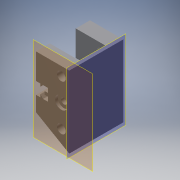
# Autodesk Inventor part: Z Slide
Saved by Autodesk Inventor 2016 (Build 200138000, 138)
## iProperties
Created: 2016-04-10
Part Number: Z Slide
Material: Generic
Document SubType Name: Modeling
Designer: Scott
Density: 1 g/cm^3
Appearance: Default
Author: Scott
Autodesk Inventor part; units mm, degrees
ref_plane "YZ Plane" through (0, 0, 0) normal (1, 0, 0) x (0, 1, 0)
ref_plane "XZ Plane" through (0, 0, 0) normal (0, 1, 0) x (-1, 0, 0)
ref_plane "XY Plane" through (0, 0, 0) normal (0, 0, 1) x (1, 0, 0)
ref_plane "Work Plane1" through (-126.0319, -64.0311, -0.0006) normal (-1, 0, 0) x (0, -1, 0)
ref_plane "Work Plane2" through (-119.6819, 11.1706, 49.5294) normal (0, 0, 1) x (0, 1, 0)
sketch "Sketch1" plane through (-119.6819, 11.1706, 49.5294) normal (0, 0, 1) x (0, 1, 0)
  line L0 (-9.2697, 67.31) -> (-9.2697, 6.35) projected
  line L1 (-9.2697, 6.35) -> (-141.1337, 6.35) projected
  line L2 (-141.1337, 6.35) -> (-141.1337, -31.75) projected
  line L3 (0, -31.75) -> (-141.1337, -31.75) projected
  line L4 (0, -31.75) -> (0, 67.31) projected
  line L5 (-9.2697, 67.31) -> (0, 67.31) projected
  line L6 (-141.1337, 6.35) -> (-105.9385, 67.31)
  line L7 (-141.1337, 6.35) -> (-70.7432, 6.35) construction
  line L8 (-105.9385, 67.31) -> (-9.2697, 67.31)
  point P0 (-11.1706, -119.6819)
  dimension "d0" = 60
  constraints: 6 end point, 2 horizontal, 1 equal length
  measures "d0" angle of L7 L6
ref_plane "Work Plane3" through (-186.9919, -129.9631, -49.5306) normal (0, 0, -1) x (0, 1, 0)
extrude "Extrusion1" add sketch "Sketch1" against normal up to surface (99.06 mm away) contours L0 L1 L6 L8
sketch "Sketch2" plane through (-186.9919, 1.9009, 49.5294) normal (0, 1, 0) x (1, 0, 0)
  line L0 (60.96, 0) -> (60.96, 99.06) projected
  line L1 (60.96, 25.3405) -> (-40.4029, 25.3405)
  line L2 (-40.4029, 25.3405) -> (-40.4029, 72.9974)
  line L3 (-40.4029, 72.9974) -> (60.96, 72.9974)
  line L4 (60.96, 72.9974) -> (60.96, 25.3405)
  point P0 (186.9919, 49.5294)
  constraints: 8 end point, 2 parallel, 1 horizontal, 1 perpendicular, 1 point on line
extrude "Extrusion2" cut sketch "Sketch2" against normal blind 61.9125
sketch "Sketch3" plane through (-119.6819, 11.1706, 49.5294) normal (0, 0, 1) x (1, 0, 0)
  line L0 (-67.31, -9.2697) -> (-67.31, -105.9385) projected
  line L1 (-67.31, -105.9385) -> (-6.35, -141.1337) projected
  line L2 (-6.35, -141.1337) -> (-6.35, -9.2697) projected
  line L3 (-6.35, -9.2697) -> (-67.31, -9.2697) projected
  circle A0 centre (-20.8167, -25.4098) radius 8
  circle A1 centre (-20.8167, -109.1654) radius 8
  line L4 (-20.8167, -25.4098) -> (-20.8167, -109.1654)
  circle A2 centre (-20.8167, -67.2876) radius 5.5
  point P0 (119.6819, -11.1706)
  dimension "d5" = 16
  dimension "d6" = 16
  dimension "d7" = 11
  constraints: 3 centre point, 2 end point, 1 midpoint, 1 vertical
  measures "d5" diameter of A0
  measures "d6" diameter of A1
  measures "d7" diameter of A2
extrude "Extrusion3" cut sketch "Sketch3" against normal blind 227.0125 contours A0 | A1 | A2 L4 | L4 A2
sketch "Sketch4" plane through (-119.6819, 11.1706, 49.5294) normal (0, 0, 1) x (1, 0, 0)
  arc A0 (-16.9332, -71.1822) -> (-24.7003, -71.1822) centre (-20.8167, -67.2876) ccw projected
  circle A1 centre (-20.8167, -67.2876) radius 11.5
  point P0 (119.6819, -11.1706)
  dimension "d10" = 23
  constraints: 1 centre point, 1 coincident
  measures "d10" diameter of A1
extrude "Extrusion4" cut sketch "Sketch4" against normal blind 5
sketch "Sketch5" plane through (-186.9919, -94.7679, 49.5294) normal (-1, 0, 0) x (0, 0, 1)
  line L0 (0, 0) -> (-99.06, 0) projected
  line L1 (-72.9974, 34.7562) -> (-72.9974, 96.6687) projected
  line L2 (-72.9974, 96.6687) -> (-99.06, 96.6687) projected
  line L3 (-99.06, 96.6687) -> (-99.06, 0) projected
  line L4 (0, 0) -> (-99.06, 0) projected
  line L5 (0, 96.6687) -> (0, 0) projected
  line L6 (0, 96.6687) -> (-25.3405, 96.6687) projected
  line L7 (-25.3405, 96.6687) -> (-25.3405, 34.7562) projected
  line L8 (-25.3405, 34.7562) -> (-72.9974, 34.7562) projected
  line L9 (-25.3405, 34.7562) -> (-25.3405, 44.1509) projected
  line L10 (-25.3405, 34.7562) -> (-72.9974, 34.7562)
  line L11 (-72.9974, 34.7562) -> (-72.9974, 22.0562)
  line L12 (-72.9974, 22.0562) -> (-25.3405, 22.0562)
  line L13 (-25.3405, 22.0562) -> (-25.3405, 34.7562)
  point P0 (-49.5294, 94.7679)
  dimension "d13" = 12.7
  constraints: 8 end point, 2 parallel, 1 horizontal, 1 perpendicular
  measures "d13" distance of L11.end L10.end
ref_plane "Work Plane4" through (-126.0319, -129.9631, -49.5306) normal (-1, 0, 0) x (0, 0, 1)
extrude "Extrusion5" cut sketch "Sketch5" against normal up to surface (60.96 mm away) contours L8 L13 L12 L11
sketch "Sketch6" plane through (-126.0319, -129.9631, 49.5294) normal (1, 0, 0) x (0, 0, -1)
  line L0 (72.9974, 57.2515) -> (72.9974, 131.864) projected
  line L1 (72.9974, 131.864) -> (99.06, 131.864) projected
  line L2 (99.06, 131.864) -> (99.06, 35.1953) projected
  line L3 (0, 35.1953) -> (99.06, 35.1953) projected
  line L4 (0, 131.864) -> (0, 35.1953) projected
  line L5 (0, 131.864) -> (25.3405, 131.864) projected
  line L6 (25.3405, 131.864) -> (25.3405, 57.2515) projected
  line L7 (25.3405, 57.2515) -> (72.9974, 57.2515) projected
  line L8 (72.9974, 131.864) -> (72.9974, 57.2515) projected
  line L9 (72.9974, 57.2515) -> (25.3405, 57.2515)
  line L10 (25.3405, 57.2515) -> (25.3405, 131.864)
  line L11 (25.3405, 131.864) -> (72.9974, 131.864)
  line L12 (72.9974, 131.864) -> (72.9974, 57.2515)
  point P0 (49.5294, 129.9631)
  constraints: 8 end point, 2 parallel, 1 horizontal, 1 perpendicular
extrude "Extrusion6" add sketch "Sketch6" against normal blind 7 contours L7 L6 L11 L0
sketch "Sketch7" plane through (-119.6819, 11.1706, 49.5294) normal (0, 0, 1) x (1, 0, 0)
  circle A0 centre (-20.8167, -67.2876) radius 11.5 projected
  circle A1 centre (-20.8167, -25.4098) radius 8 projected
  circle A2 centre (-20.8167, -109.1654) radius 8 projected
  line L0 (-67.31, -9.2697) -> (-67.31, -105.9385) projected
  line L1 (-67.31, -105.9385) -> (-6.35, -141.1337) projected
  line L2 (-6.35, -141.1337) -> (-6.35, -9.2697) projected
  line L3 (-6.35, -9.2697) -> (-67.31, -9.2697) projected
  line L4 (-45.32, -56.2876) -> (-67.32, -56.2876)
  line L5 (-67.32, -56.2876) -> (-67.32, -78.2876)
  line L6 (-67.32, -78.2876) -> (-45.32, -78.2876)
  line L7 (-45.32, -78.2876) -> (-45.32, -56.2876)
  line L8 (-45.32, -56.2876) -> (-67.32, -78.2876) construction
  line L9 (-67.32, -56.2876) -> (-45.32, -78.2876) construction
  point P0 (119.6819, -11.1706)
  point P1 (-56.32, -67.2876)
  dimension "d18" = 22
  dimension "d19" = 22
  constraints: 12 end point, 2 midpoint, 2 parallel, 1 horizontal, 1 perpendicular
  measures "d18" distance of L6.end L5.end
  measures "d19" distance of L5.end L4.end
extrude "Extrusion7" cut sketch "Sketch7" against normal blind 508 contours L4 L7 L6 L0 | L0 L6 L5 L4
sketch "Sketch8" plane through (-119.6819, 11.1706, 49.5294) normal (0, 0, 1) x (1, 0, 0)
  line L0 (-67.31, -56.2876) -> (-45.32, -56.2876) projected
  line L1 (-45.32, -56.2876) -> (-45.32, -78.2876) projected
  line L2 (-45.32, -78.2876) -> (-67.31, -78.2876) projected
  line L3 (-67.31, -78.2876) -> (-67.31, -105.9385) projected
  line L4 (-67.31, -105.9385) -> (-6.35, -141.1337) projected
  line L5 (-6.35, -141.1337) -> (-6.35, -9.2697) projected
  line L6 (-6.35, -9.2697) -> (-67.31, -9.2697) projected
  line L7 (-67.31, -9.2697) -> (-67.31, -56.2876) projected
  circle A0 centre (-20.8167, -109.1654) radius 8 projected
  circle A1 centre (-20.8167, -25.4098) radius 8 projected
  circle A2 centre (-20.8167, -67.2876) radius 11.5 projected
  line L8 (-45.32, -67.2876) -> (-48.32, -67.2876)
  line L9 (-51.32, -64.2876) -> (-45.32, -64.2876)
  line L10 (-45.32, -64.2876) -> (-45.32, -70.2876)
  line L11 (-45.32, -70.2876) -> (-51.32, -70.2876)
  line L12 (-51.32, -70.2876) -> (-51.32, -64.2876)
  line L13 (-51.32, -64.2876) -> (-45.32, -70.2876) construction
  line L14 (-45.32, -64.2876) -> (-51.32, -70.2876) construction
  line L15 (-45.32, -78.2876) -> (-45.32, -56.2876) projected
  line L16 (-45.32, -78.2876) -> (-56.315, -78.2876)
  line L17 (-67.31, -78.2876) -> (-45.32, -78.2876) projected
  line L18 (-56.315, -78.2876) -> (-59.315, -78.2876)
  line L19 (-59.315, -78.2876) -> (-59.315, -73.2876)
  line L20 (-59.315, -73.2876) -> (-54.315, -78.2876)
  line L21 (-59.315, -56.2876) -> (-59.315, -61.2876)
  line L22 (-59.315, -61.2876) -> (-54.315, -56.2876)
  line L23 (-45.32, -56.2876) -> (-67.31, -56.2876) projected
  line L24 (-59.315, -56.2876) -> (-54.315, -56.2876)
  point P0 (119.6819, -11.1706)
  dimension "d22" = 3
  dimension "d23" = 6
  dimension "d24" = 6
  dimension "d25" = 3
  dimension "d26" = 5
  dimension "d27" = 5
  constraints: 28 end point, 4 midpoint, 4 point on line, 2 horizontal, 2 parallel, 2 perpendicular, 1 collinear, 1 vertical
  measures "d22" distance of L8.start L8.end
  measures "d23" distance of L10.end L11.end
  measures "d24" distance of L9.end L10.end
  measures "d25" distance of L16.end L18.end
  measures "d26" distance of L18.end L19.end
  measures "d27" distance of L21.start L21.end
extrude "Extrusion8" add sketch "Sketch8" against normal up to surface (99.06 mm away) contours L0 L22 L21 | L1 L11 L12 L9 | L19 L20 L2
sketch "Sketch10" plane through (-186.9919, -72.7116, 24.1889) normal (0, 1, 0) x (1, 0, 0)
  line L0 (0, 47.6568) -> (53.96, 47.6568) projected
  line L1 (0, 0) -> (0, 47.6568) projected
  line L2 (0, 0) -> (53.96, 0) projected
  line L3 (53.96, 0) -> (53.96, 47.6568) projected
  point P0 (186.9919, 24.1889)
extrude "Extrusion9" cut sketch "Sketch10" along normal blind 508
body "Solid1"
